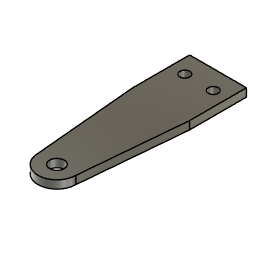
Fork End v21 (Autodesk Fusion 360 design; units mm, degrees)
Autodesk Fusion 360 part; units mm, degrees
sketch "Main" plane through (0, 0, 0) normal (0, 0, 1) x (1, 0, 0)
  line L0 (-6, 34) -> (6, 34)
  arc A0 (-3.9956, -0.1866) -> (4, 0) centre (0, 0) ccw
  line L1 (-6, 22) -> (-3.9956, -0.1866)
  circle A1 centre (0, 0) radius 1.55
  line L2 (6, 34) -> (6, 22)
  line L3 (-6, 34) -> (-6, 22)
  line L4 (6, 22) -> (4, 0)
  dimension "d1" = 4
  dimension "d2" = 3.1
  dimension "d3" = 12
  dimension "d4" = 6
  dimension "d5" = 12
  dimension "d6" = 12
  dimension "d7" = 34
  constraint horizontal L0
  constraint coincident A0.centre A1.centre
  constraint concentric A0 A1
  constraint perpendicular L0 L2
  constraint perpendicular L0 L3
  constraint coincident L1.start L3.end
  constraint horizontal A0.end A0.centre
  measures "d1" radius of A0
  measures "d2" diameter of A1
  measures "d3" distance of L0.start L0.end
  measures "d4" horizontal distance of L0.end A0.centre
  measures "d5" distance of L0.end L2.end
  measures "d6" distance of L0.start L1.start
  measures "d7" distance of L0 A0.centre
extrude "Extrude1" add sketch "Main" along normal blind 1.7
sketch "Holes" plane through (0, 0, 1.7) normal (0, 0, 1) x (-1, 0, 0)
  circle A0 centre (0, 0) radius 1.55
  line L0 (6, -34) -> (6, -22)
  line L1 (6, -22) -> (3.9956, 0.1866)
  arc A1 (3.9956, 0.1866) -> (-4, 0) centre (0, 0) ccw
  line L2 (-4, 0) -> (-6, -22)
  line L3 (-6, -22) -> (-6, -34)
  line L4 (-6, -34) -> (6, -34)
  line L5 (6, -30) -> (-6, -30) construction
  circle A2 centre (3, -30) radius 1.05
  circle A3 centre (-3, -30) radius 1.05
  dimension "d10" = 4
  dimension "d11" = 2.1
  dimension "d12" = 2.1
  dimension "d13" = 6
  dimension "d14" = 3
  constraint coincident L0 L5.start
  constraint coincident L3 L5.end
  constraint perpendicular L3 L5
  constraint coincident L5 A2.centre
  constraint coincident L5 A3.centre
  measures "d10" distance of L4 L5
  measures "d11" diameter of A2
  measures "d12" diameter of A3
  measures "d13" distance of A2.centre A3.centre
  measures "d14" distance of L0 A2.centre
extrude "Extrude2" cut sketch "Holes" against normal up to surface (1.7 mm away) contours A2 | A3
